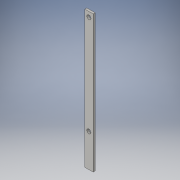
# Autodesk Inventor part: grabber articulation arms
Saved by Autodesk Inventor 2016 SP2 (Build 200236200, 236)
## iProperties
Created: 2018-02-13
Part Number: grabber articulation arms
Material: Generic
Document SubType Name: Modeling
Designer: CAD
Density: 1 g/cm^3
Appearance: Default
Author: CAD
Autodesk Inventor part; units mm, degrees
ref_plane "YZ Plane" through (0, 0, 0) normal (1, 0, 0) x (0, 1, 0)
ref_plane "XZ Plane" through (0, 0, 0) normal (0, 1, 0) x (-1, 0, 0)
ref_plane "XY Plane" through (0, 0, 0) normal (0, 0, 1) x (1, 0, 0)
sketch "Sketch1" plane through (0, 0, 0) normal (0, 1, 0) x (-1, 0, 0)
  line L0 (0, 0) -> (12.7, 0)
  line L1 (0, 0) -> (0, -3.175)
  line L2 (12.7, 0) -> (12.7, -3.175)
  line L3 (12.7, -3.175) -> (0, -3.175)
  dimension "d2" = 3.175
  dimension "d3" = 12.7
  constraints: 8 end point, 2 vertical, 1 horizontal, 1 perpendicular
  measures "d2" distance of L0.start L1.end
  measures "d3" distance of L0.start L0.end
extrude "Extrusion1" add sketch "Sketch1" along normal blind 209.55
sketch "Sketch2" plane through (-12.7, 0, 0) normal (0, 0, 1) x (1, 0, 0)
  line L0 (0, 209.55) -> (12.7, 209.55) projected
  line L1 (0, 0) -> (0, 209.55) projected
  line L2 (12.7, 0) -> (0, 0) projected
  point P0 (6.35, 201.93)
  point P1 (6.35, 50.8)
  dimension "d6" = 7.62
  dimension "d7" = 6.35
  dimension "d8" = 50.8
  dimension "d9" = 6.35
  measures "d6" distance from line of L0 point (6.35, 201.93)
  measures "d7" distance from line of L1 point (6.35, 201.93)
  measures "d8" distance from line of L2 point (6.35, 50.8)
  measures "d9" distance from line of point (6.35, 50.8) L1
hole "Hole1" at (-6.35, 201.93, 0) at (-6.35, 50.8, 0) direction (0, 0, -1) diameter 6.35 end through all
body "Solid1"
